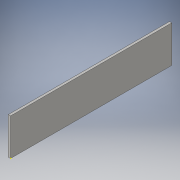
# Autodesk Inventor part: DriveTrainPlate
Saved by Autodesk Inventor 2016 (Build 200138000, 138)
## iProperties
Created: 2016-09-21
Part Number: DriveTrainPlate
Material: Generic
Document SubType Name: Modeling
Designer: RoboticsUser
Density: 1 g/cm^3
Appearance: Default
Author: RoboticsUser
Autodesk Inventor part; units mm, degrees
ref_plane "YZ Plane" through (0, 0, 0) normal (1, 0, 0) x (0, 1, 0)
ref_plane "XZ Plane" through (0, 0, 0) normal (0, 1, 0) x (-1, 0, 0)
ref_plane "XY Plane" through (0, 0, 0) normal (0, 0, 1) x (1, 0, 0)
sketch "Sketch1" plane through (0, 0, 0) normal (1, 0, 0) x (0, 1, 0)
  line L0 (444.5, 0) -> (444.5, -2.1042)
  line L1 (0, -2.1042) -> (0, 0)
  line L2 (0, -74.1174) -> (0, -66.8433)
  line L3 (0, 0) -> (101.6, 0)
  line L4 (101.6, 0) -> (101.6, -444.5)
  line L5 (101.6, -444.5) -> (0, -444.5)
  line L6 (0, -444.5) -> (0, 0)
  point P0 (38.1, -50.8)
  point P1 (38.1, -393.7)
  dimension "d2" = 101.6
  dimension "d3" = 444.5
  dimension "d4" = 50.8
  dimension "d5" = 38.1
  dimension "d6" = 50.8
  dimension "d7" = 38.1
  constraints: 14 end point, 3 parallel, 1 horizontal, 1 perpendicular, 1 point on line
  measures "d2" distance of L4.end L5.end
  measures "d3" distance of L3.end L4.end
  measures "d4" distance from line of L3 point (38.1, -50.8)
  measures "d5" distance from line of L6 point (38.1, -50.8)
  measures "d6" distance from line of L5 point (38.1, -393.7)
  measures "d7" distance from line of L6 point (38.1, -393.7)
extrude "Extrusion1" add sketch "Sketch1" along normal blind 6.35
sketch "Sketch3" plane through (6.35, 0, 0) normal (1, 0, 0) x (0, 0, -1)
  point P0 (0, 0)
body "Solid1"
